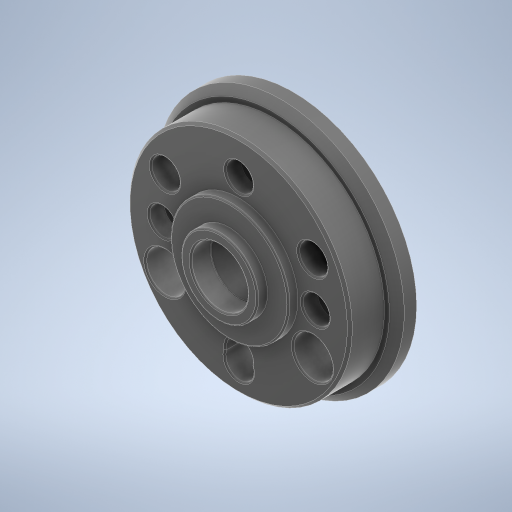
# Autodesk Inventor part: motor_main_drive_mount
Saved by Autodesk Inventor 2023 (Build 270158000, 158)
## iProperties
Created: 2023-11-23
Part Number: motor_main_drive_mount
Material: Acetal Resin, Black
Document SubType Name: Modeling
Designer: aaron
Density: 1.425 g/cm^3
Appearance: Smooth - Black
Author: aaron
Autodesk Inventor part; units mm, degrees
ref_plane "YZ Plane" through (0, 0, 0) normal (1, 0, 0) x (0, 1, 0)
ref_plane "XZ Plane" through (0, 0, 0) normal (0, 1, 0) x (-1, 0, 0)
ref_plane "XY Plane" through (0, 0, 0) normal (0, 0, 1) x (1, 0, 0)
sketch "Sketch1" plane through (0, 0, 0) normal (0, 0, 1) x (1, 0, 0)
  circle A0 centre (0, 0) radius 15.5
  circle A1 centre (0, 15.5) radius 1.55
  circle A2 centre (-15.5, 0) radius 1.55
  circle A3 centre (0, -15.5) radius 1.55
  circle A4 centre (15.5, 0) radius 1.55
  circle A5 centre (0, 0) radius 25
  circle A6 centre (0, 0) radius 21.985
  circle A7 centre (0, 0) radius 17.235
  circle A8 centre (0, 17.235) radius 2.9
  circle A9 centre (-14.9259, 8.6175) radius 2.9
  circle A10 centre (-14.9259, -8.6175) radius 2.9
  circle A11 centre (0, -17.235) radius 2.9
  circle A12 centre (14.9259, -8.6175) radius 2.9
  circle A13 centre (14.9259, 8.6175) radius 2.9
  dimension "d0" = 31
  dimension "d3" = 360
  dimension "d5" = 3.1
  dimension "d7" = 50
  dimension "d8" = 43.97
  dimension "d9" = 4.75
  dimension "d10" = 5.8
  dimension "d13" = 360
  constraints: 12 centre point, 3 coincident, 2 vertical alignment, 26 other
  measures "d5" diameter of A1
  measures "d7" diameter of A5
  measures "d8" diameter of A6
  measures "d10" diameter of A8
extrude "Extrusion1" add sketch "Sketch1" against normal blind 11 contours A4 A0 A12 A11 A3 A10 A2 A9 A8 A1 A13 | A0 A13 A7 A12 A4 | A12 A7 A0 | A0 A12 | A0 A8 A7 A13 | A12 A7 A11 A0 | A12 A7 | A8 A1 A0 | A0 A1 A8 A7 | A11 A7 A0 A3 | A0 A3 A11 | A7 A8 | A11 A7 | A1 A8 A0 | A8 A0 A9 A7 | A0 A11 A3 | A7 A10 A0 A11 | A10 A7 | A7 A10 A0 | A9 A0 A2 A10 A7 | A0 A10 | A5 | A6 picked at (1.7337, 15.2043) picked at (1.7337, -15.2043) picked at (-1.7337, 15.2043) picked at (-1.7337, -15.2043)
sketch "Sketch2" plane through (0, 0, 0) normal (0, 0, 1) x (1, 0, 0)
  circle A0 centre (0, 15.5) radius 1.55 projected
  circle A1 centre (0, 15.5) radius 3.4395
  circle A2 centre (14.9259, 8.6175) radius 2.9
  circle A3 centre (0, 17.235) radius 2.9
  circle A4 centre (-14.9259, 8.6175) radius 2.9
  circle A5 centre (-14.9259, -8.6175) radius 2.9
  circle A6 centre (0, -17.235) radius 2.9
  circle A7 centre (14.9259, -8.6175) radius 2.9
  point P0 (0, 0)
  dimension "d19" = 360
  constraints: 7 centre point, 1 coincident, 13 other
extrude "Extrusion2" cut sketch "Sketch2" against normal blind 6.1 contours A6
sketch "Sketch3" plane through (0, 0, 0) normal (0, 0, 1) x (1, 0, 0)
  circle A0 centre (0, 15.5) radius 1.55 projected
  circle A1 centre (0, 15.5) radius 2.75
  circle A2 centre (-15.5, 0) radius 2.75
  circle A3 centre (0, -15.5) radius 2.75
  circle A4 centre (15.5, 0) radius 2.75
  point P0 (0, 0)
  dimension "d23" = 5.5
  dimension "d26" = 360
  constraints: 4 centre point, 1 coincident, 9 other
  measures "d23" diameter of A1
extrude "Extrusion3" cut sketch "Sketch3" against normal blind 3.2 contours A0 | A1 | A2 | A3 | A4
sketch "Sketch4" plane through (0, 0, 0) normal (0, 0, 1) x (1, 0, 0)
  arc A0 (2.6784, -16.1233) -> (-2.6784, -16.1233) centre (0, -15.5) ccw projected
  circle A1 centre (0, -15.5) radius 2.75
  point P0 (0, 0)
  point P1 (-2.6784, -16.1233)
  point P2 (2.6784, -16.1233)
  constraints: 1 centre point, 1 coincident
extrude "Extrusion4" cut sketch "Sketch4" against normal blind 9.3
sketch "Sketch5" plane through (0, 0, 0) normal (0, 0, 1) x (1, 0, 0)
  circle A0 centre (0, 0) radius 1.55
  dimension "d32" = 3.1
  constraints: 1 centre point, 1 coincident
  measures "d32" diameter of A0
extrude "Extrusion5" cut sketch "Sketch5" against normal through all
sketch "Sketch6" plane through (0, 0, 0) normal (0, 0, 1) x (1, 0, 0)
  circle A0 centre (14.9259, 8.6175) radius 2.9 projected
  circle A1 centre (14.9259, 8.6175) radius 3.99
  circle A2 centre (0, 17.235) radius 3.99
  circle A3 centre (-14.9259, 8.6175) radius 3.99
  circle A4 centre (-14.9259, -8.6175) radius 3.99
  circle A5 centre (0, -17.235) radius 3.99
  circle A6 centre (14.9259, -8.6175) radius 3.99
  point P0 (0, 0)
  dimension "d35" = 7.98
  dimension "d38" = 360
  constraints: 6 centre point, 1 coincident, 13 other
  measures "d35" diameter of A1
extrude "Extrusion6" cut sketch "Sketch6" against normal blind 7 contours A4 | A6
sketch "Sketch7" plane through (0, 0, 0) normal (0, 0, 1) x (1, 0, 0)
  circle A0 centre (0, 0) radius 7.75
  circle A1 centre (0, 0) radius 5.75
  dimension "d42" = 15.5
  dimension "d43" = 2
  constraints: 2 centre point, 1 coincident
  measures "d42" diameter of A0
  measures "d43" radial gap between concentric circles of A0 A1
extrude "Extrusion7" add sketch "Sketch7" along normal blind 4
sketch "Sketch8" plane through (0, 0, 0) normal (0, 0, 1) x (1, 0, 0)
  circle A0 centre (0, 0) radius 5.75 projected
  circle A1 centre (0, 0) radius 11.975
  circle A2 centre (0, 0) radius 7.75
  dimension "d46" = 23.95
  constraints: 2 centre point, 2 coincident
  measures "d46" diameter of A1
extrude "Extrusion8" add sketch "Sketch8" along normal blind 1.9 contours A1
chamfer "Chamfer1" distance 3 angle 45 1 edges at (-25, 0, 0)
chamfer "Chamfer2" distance 4 angle 45 1 edges at (-1.55, 0, 0)
fillet "Fillet1" radius 0.3 12 edges at (-5.75, 0, 4) (-7.75, 0, 4) (-11.975, 0, 1.9) (10.9359, -8.6175, 0) (12.75, 0, 0) (12.0259, 8.6175, 0) (-2.75, 15.5, 0) (-17.8259, 8.6175, 0) (-18.25, 0, 0) (-18.9159, -8.6175, 0) (0, -20.135, 0) (0, -12.75, 0)
sketch "Sketch9" plane through (0, 0, 0) normal (0, 0, 1) x (1, 0, 0)
  circle A0 centre (0, 0) radius 1.55 projected
  circle A1 centre (0, 0) radius 22.5
  circle A2 centre (0, 0) radius 32.9139
  dimension "d56" = 45
  constraints: 2 centre point, 2 coincident
  measures "d56" diameter of A1
extrude "Extrusion9" cut sketch "Sketch9" against normal blind 7 contours A2
chamfer "Chamfer3" distance 1.5 angle 45 1 edges at (-25, 0, -7)
body "Solid1"
